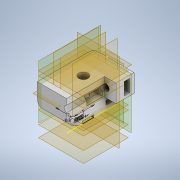
# Autodesk Inventor part: Encoder_Mount2
Saved by Autodesk Inventor 2022 (Build 260153000, 153)
## iProperties
Created: 2024-04-29
Part Number: Encoder_Mount2
Material: Generic
Document SubType Name: Modeling
Designer: Gotham City
Density: 1 g/cm^3
Appearance: Default
Author: Gotham City
Autodesk Inventor part; units mm, degrees
ref_plane "Alu_Top" through (0, 0, 0) normal (0, 1, 0) x (-1, 0, 0)
ref_plane "Strip" through (0, -20.8, 0) normal (0, 1, 0) x (-1, 0, 0)
ref_plane "Alu_Bottom" through (0, -2, 0) normal (0, 1, 0) x (-1, 0, 0)
ref_plane "EncoderPCB_Top" through (0, -25.8, 0) normal (0, 1, 0) x (-1, 0, 0)
ref_plane "Strip_V_End" through (5, 0, 0) normal (1, 0, 0) x (0, 1, 0)
ref_plane "Strip_V_Start" through (0, 0, 0) normal (1, 0, 0) x (0, 1, 0)
ref_plane "Encoder_PCB_Bottom" through (0, -15.2, 0) normal (0, 1, 0) x (-1, 0, 0)
ref_plane "Encoder_ScrewMount_V" through (-3.5, 0, 0) normal (1, 0, 0) x (0, 1, 0)
sketch "Sketch5" plane through (0, 0, 0) normal (0, 0, 1) x (1, 0, 0)
  line L0 (-7, -18.8) -> (5, -18.8)
  line L1 (5, -18.8) -> (5, -25.8)
  line L2 (5, -25.8) -> (-7, -25.8)
  line L3 (-7, -25.8) -> (-7, -18.8)
  line L4 (5, 5.06) -> (5, -30.36) construction
  line L5 (-9.4, -25.8) -> (7.4, -25.8) construction
  point P0 (0, 0)
  dimension "d10" = 12
  dimension "d11" = 7
  constraints: 8 end point, 2 parallel, 2 point on line, 1 horizontal, 1 perpendicular
  measures "d10" distance of L0.start L0.end
  measures "d11" distance of L0.end L1.end
extrude "Extrusion1" add sketch "Sketch5" along normal mid plane 7
sketch "Sketch6" plane through (-7, -25.8, 3.5) normal (0, -1, 0) x (1, 0, 0)
  line L0 (0, -12.5) -> (6.5, -12.5)
  line L1 (6.5, -12.5) -> (6.5, 5.5)
  line L2 (6.5, 5.5) -> (0, 5.5)
  line L3 (0, 5.5) -> (0, -12.5)
  line L4 (-2.4, -3.5) -> (14.4, -3.5) construction
  line L5 (3.5, 182.4494) -> (3.5, -189.4494) construction
  circle A0 centre (3.5, -10.5) radius 1
  line L6 (3.5, -189.4494) -> (3.5, 182.4494) construction
  circle A1 centre (3.5, 3.5) radius 1
  point P0 (7, -3.5)
  point P1 (0, -7)
  dimension "d14" = 18
  dimension "d15" = 6.5
  dimension "d16" = 14
  dimension "d17" = 2
  constraints: 10 end point, 3 point on line, 3 symmetric about line, 2 centre point, 2 parallel, 1 horizontal, 1 perpendicular, 2 other
  measures "d14" distance of L2.end L0.start
  measures "d15" distance of L0.start L0.end
  measures "d16" distance of A1.centre A0.centre
  measures "d17" diameter of A0
extrude "Extrusion2" add sketch "Sketch6" against normal up to surface (10.6 mm away)
sketch "Sketch4" plane through (0, 0, 0) normal (0, 0, 1) x (1, 0, 0)
  line L0 (-19.2812, -2) -> (9.0469, -2) construction
  line L1 (-8, -2) -> (5, -2)
  line L2 (5, -2) -> (5, -15.2)
  line L3 (5, -15.2) -> (-8, -15.2)
  line L4 (-8, -15.2) -> (-8, -2)
  line L5 (0, 3.75) -> (0, -22.5) construction
  line L6 (-8, -2) -> (-15.2344, -2) construction
  line L7 (-15.2344, -2) -> (-15.2344, -18.75) construction
  line L8 (-15.2344, -18.75) -> (-8, -18.75) construction
  line L9 (-8, -18.75) -> (-8, -2) construction
  line L10 (-19.2812, -15.2) -> (9.0469, -15.2) construction
  point P0 (0, 0)
  dimension "d54" = 5
  dimension "d55" = 8
  constraints: 16 end point, 4 parallel, 2 horizontal, 2 perpendicular, 2 point on line
  measures "d54" distance between parallel lines of L5 L2
  measures "d55" distance between parallel lines of L4 L5
extrude "Extrusion3" add sketch "Sketch4" along normal mid plane 25 separate body
ref_plane "SideA" through (0, 0, -12.5) normal (0, 0, -1) x (-1, 0, 0)
sketch "Sketch19" plane through (0, 0, -12.5) normal (0, 0, -1) x (-1, 0, 0)
  line L0 (-5, -2) -> (8, -2) projected
  line L1 (-5, -2) -> (-10, -2)
  line L2 (-10, -2) -> (-10, -10)
  line L3 (-10, -10) -> (-5, -10)
  line L4 (-5, -10) -> (-5, -2)
  point P0 (0, 0)
  dimension "d73" = 8
  dimension "d74" = 5
  constraints: 8 end point, 2 parallel, 1 horizontal, 1 perpendicular
  measures "d73" distance of L1.end L2.end
  measures "d74" distance of L0.start L1.end
extrude "Extrusion10" add sketch "Sketch19" against normal blind 8
sketch "Sketch7" plane through (0, 0, 0) normal (1, 0, 0) x (0, 1, 0)
  line L0 (-17.8, -3.5) -> (-17.8, 3.5) projected
  line L1 (-15.2, -12.5) -> (-15.2, 12.5) projected
  line L2 (-17.8, 3.5) -> (-15.2, 3.5)
  line L3 (-15.2, 3.5) -> (-15.2, -3.5)
  line L4 (-15.2, -3.5) -> (-17.8, -3.5)
  line L5 (-17.8, -3.5) -> (-17.8, 3.5)
  point P0 (0, 0)
  constraints: 8 end point, 2 parallel, 1 horizontal, 1 perpendicular, 1 point on line
extrude "Extrusion4" [suppressed]
sketch "Sketch8" plane through (0, -15.2, 0) normal (0, 1, 0) x (-1, 0, 0)
  circle A0 centre (3.5, 7) radius 1 projected
  circle A1 centre (3.5, -7) radius 1 projected
  point P0 (0, 0)
hole "Hole1" at (-3.5, -15.2, 7) at (-3.5, -15.2, -7) direction (0, 1, 0) diameter 2.1 depth 10 tip angle 118 clearance for "Socket Head Cap Screw ISO 4762" size "M2" standard "ISO"
ref_plane "Nut12" through (0, -13.2, 0) normal (0, 1, 0) x (-1, 0, 0)
sketch "Sketch10" plane through (0, -13.2, 0) normal (0, 1, 0) x (-1, 0, 0)
  circle A0 centre (3.5, 7) radius 1 construction
  line L0 (4.6691, 4.975) -> (2.3309, 4.975)
  line L1 (2.3309, 4.975) -> (1.1617, 7) construction
  line L2 (1.1617, 7) -> (2.3309, 9.025) construction
  line L3 (2.3309, 9.025) -> (4.6691, 9.025)
  line L4 (4.6691, 9.025) -> (5.8383, 7)
  line L5 (5.8383, 7) -> (4.6691, 4.975)
  line L6 (2.3309, 4.975) -> (-10, 4.975)
  line L7 (2.3309, 9.025) -> (-10, 9.025)
  line L8 (-10, 9.025) -> (-10, 4.975)
  line L9 (-10, -12.5) -> (-10, -4.5) projected
  point P0 (0, 0)
  dimension "d32" = 4.05
  constraints: 18 end point, 3 horizontal, 1 coincident, 1 perpendicular, 1 point on line, 13 other
  measures "d32" distance between parallel lines of L0 L3
extrude "Extrusion5" cut sketch "Sketch10" along normal blind 1.63
mirror "Mirror1" about plane through (0, 0, 0) normal (0, 0, 1) of "Extrusion5"
sketch "Sketch11" plane through (-8, -2, 12.5) normal (0, 1, 0) x (1, 0, 0)
  point P0 (8, 12.5)
  point P1 (8, 12.5)
  constraints: 1 coincident
hole "Hole2" at (0, -2, 0) direction (0, -1, 0) diameter 4.1 depth 8 tip angle 118 clearance for "Socket Head Cap Screw ISO 4762" size "M4" standard "ISO"
ref_plane "Nut3" through (-8, -6, 12.5) normal (0, 1, 0) x (1, 0, 0)
sketch "Sketch12" plane through (-8, -6, 12.5) normal (0, 1, 0) x (1, 0, 0)
  line L0 (3.9297, 12.5) -> (5.9648, 16.025)
  line L1 (5.9648, 16.025) -> (10.0352, 16.025)
  line L2 (10.0352, 16.025) -> (12.0703, 12.5) construction
  line L3 (12.0703, 12.5) -> (10.0352, 8.975) construction
  line L4 (10.0352, 8.975) -> (5.9648, 8.975)
  line L5 (5.9648, 8.975) -> (3.9297, 12.5)
  line L6 (10.0352, 16.025) -> (13, 16.025)
  line L7 (13, 17) -> (13, 0) projected
  line L8 (10.0352, 8.975) -> (13, 8.975)
  point P0 (8, 12.5)
  point P1 (8, 12.5)
  point P2 (13, 25)
  dimension "d45" = 7.05
  constraints: 16 end point, 2 horizontal, 2 point on line, 1 coincident, 1 parallel, 13 other
  measures "d45" distance between parallel lines of L1 L4
extrude "Extrusion6" cut sketch "Sketch12" against normal blind 3.25
sketch "Sketch13" plane through (0, 0, 0) normal (0, 0, 1) x (1, 0, 0)
  line L0 (-3, -19.8) -> (8, -19.8)
  line L1 (8, -19.8) -> (8, -21.8)
  line L2 (8, -21.8) -> (-3, -21.8)
  line L3 (-3, -21.8) -> (-3, -19.8)
  line L4 (0, 4.26) -> (0, -25.56) construction
  line L5 (5, 4.26) -> (5, -25.56) construction
  line L6 (-5.2, -20.8) -> (10.2, -20.8) construction
  point P0 (0, 0)
  dimension "d46" = 3
  dimension "d47" = 3
  dimension "d48" = 1
  dimension "d49" = 1
  constraints: 8 end point, 2 parallel, 1 horizontal, 1 perpendicular
  measures "d46" distance between parallel lines of L4 L3
  measures "d47" distance between parallel lines of L1 L5
  measures "d48" distance between parallel lines of L6 L0
  measures "d49" distance between parallel lines of L6 L2
extrude "Extrusion7" [suppressed]
ref_plane "EndstopScrew" through (0, -4.5, 0) normal (0, 1, 0) x (-1, 0, 0)
sketch "Sketch17" plane through (0, 0, -12.5) normal (0, 0, -1) x (-1, 0, 0)
  line L0 (-8.2, -6) -> (10.7, -6) projected
  point P0 (0, 0)
  point P1 (-5.5, -6)
  dimension "d60" = 5.5
  constraints: 1 point on line
  measures "d60" horizontal distance of point (0, 0) point (-5.5, -6)
hole "Hole3" at (5.5, -6, -12.5) direction (0, 0, 1) diameter 3 end through all clearance for "Socket Head Cap Screw ISO 4762" size "M3" standard "ISO"
ref_plane "Work Plane13" through (0, 0, -10.5) normal (0, 0, -1) x (-1, 0, 0)
sketch "Sketch18" plane through (0, 0, -10.5) normal (0, 0, -1) x (-1, 0, 0)
  circle A0 centre (-5.5, -6) radius 1.5 projected
  line L0 (-3.8979, -3.225) -> (-2.2957, -6)
  line L1 (-2.2957, -6) -> (-3.8979, -8.775)
  line L2 (-3.8979, -8.775) -> (-7.1021, -8.775)
  line L3 (-7.1021, -8.775) -> (-8.7043, -6) construction
  line L4 (-8.7043, -6) -> (-7.1021, -3.225) construction
  line L5 (-7.1021, -3.225) -> (-3.8979, -3.225)
  line L6 (-7.1021, -3.225) -> (-10, -3.225)
  line L7 (-7.1021, -8.775) -> (-10, -8.775)
  line L8 (-10, -10) -> (-10, -2) projected
  point P0 (0, 0)
  point P1 (-13, -14.8)
  point P2 (-10, -2)
  dimension "d69" = 5.55
  constraints: 16 end point, 4 horizontal, 2 coincident, 1 parallel, 16 other
  measures "d69" distance between parallel lines of L2 L5
extrude "Extrusion9" cut sketch "Sketch18" against normal blind 2.35
fillet "Fillet1" [suppressed]
thicken "Thicken1" [suppressed]
sketch "Sketch22" plane through (-3, -22.8, 3.5) normal (0, -1, 0) x (1, 0, 0)
  line L0 (-5, -16) -> (13, -16) projected
  line L1 (8, 9) -> (4, 9)
  line L2 (4, 9) -> (4, -16)
  line L3 (4, -16) -> (8, -16)
  line L4 (8, -16) -> (8, 9)
  line L5 (-5, 9) -> (-5, 0.1) projected
  circle A0 centre (-0.5, 3.5) radius 1.05 projected
  point P0 (3, -3.5)
  point P1 (8, 9)
  dimension "d84" = 4.5
  dimension "d85" = 4.5
  constraints: 8 end point, 2 parallel, 1 coincident, 1 horizontal, 1 midpoint, 1 perpendicular
  measures "d84" distance from line of L5 A0.centre
  measures "d85" distance from line of L2 A0.centre
extrude "Extrusion11" [suppressed]
ref_plane "Work Plane16" through (0, 0, -5) normal (0, 0, 1) x (1, 0, 0)
sketch "Sketch23" plane through (0, 0, -10.5) normal (0, 0, -1) x (-1, 0, 0)
  point P0 (0, 0)
sketch "Sketch24" plane through (-8, -15.2, 12.5) normal (-1, 0, 0) x (0, 0, 1)
  line L0 (-17.5, 20.36) -> (-17.5, -15.76) construction
  line L1 (-22, 5.2) -> (-13, 5.2) construction
  line L2 (-22, 4.15) -> (-13, 4.15)
  line L3 (-13, 6.25) -> (-22, 6.25)
  arc A0 (-22, 6.25) -> (-22, 4.15) centre (-22, 5.2) ccw
  arc A1 (-13, 4.15) -> (-13, 6.25) centre (-13, 5.2) ccw
  line L4 (-25, 13.2) -> (0, 13.2) projected
  point P0 (-12.5, 15.2)
  point P1 (-17.5, 5.2)
  dimension "d91" = 9
  dimension "d92" = 2.1
  dimension "d93" = 8
  constraints: 8 end point, 4 point on circle, 4 tangent, 2 centre point, 1 midpoint, 1 parallel, 1 perpendicular, 1 point on line
  measures "d91" distance of L1.start L1.end
  measures "d92" distance between parallel lines of L3 L2
  measures "d93" distance between parallel lines of L4 L1
ref_plane "Work Plane17" through (-6, -15.2, 12.5) normal (-1, 0, 0) x (0, 0, 1)
sketch "Sketch25" plane through (-6, -15.2, 12.5) normal (-1, 0, 0) x (0, 0, 1)
  line L0 (-25, 0) -> (-25, 13.2) projected
  line L1 (-25, 7.25) -> (-10.6329, 7.25)
  line L2 (-10.6329, 7.25) -> (-10.6329, 3.15)
  line L3 (-10.6329, 3.15) -> (-25, 3.15)
  line L4 (-25, 3.15) -> (-25, 7.25)
  line L5 (-25, 5.2) -> (-17, 5.2) projected
  line L6 (0, 0) -> (-25, 0) projected
  line L7 (0, 13.2) -> (0, 0) projected
  line L8 (-25, 13.2) -> (0, 13.2) projected
  line L9 (-25, 0) -> (-25, 13.2) projected
  line L10 (-11.8164, 3.15) -> (-14.1836, 3.15)
  line L11 (-14.1836, 3.15) -> (-15.3671, 5.2) construction
  line L12 (-15.3671, 5.2) -> (-14.1836, 7.25) construction
  line L13 (-14.1836, 7.25) -> (-11.8164, 7.25)
  line L14 (-11.8164, 7.25) -> (-10.6329, 5.2) construction
  line L15 (-10.6329, 5.2) -> (-11.8164, 3.15) construction
  point P0 (-12.5, 15.2)
  point P1 (-13, 5.2)
  point P2 (-13, 5.2)
  dimension "d95" = 4.1
  constraints: 20 end point, 2 horizontal, 2 parallel, 2 point on line, 1 coincident, 1 midpoint, 1 perpendicular, 14 other
  measures "d95" distance of L1.end L2.end
extrude "Extrusion12" [suppressed]
extrude "Extrusion13" [suppressed]
sketch "Sketch26" plane through (-8, -15.2, 12.5) normal (0, -1, 0) x (1, 0, 0)
  line L0 (8, -8) -> (1, -8)
  line L1 (1, -8) -> (1, -17)
  line L2 (1, -17) -> (8, -17)
  line L3 (8, -17) -> (8, -8)
  line L4 (4.5, -5.5) -> (4.5, -8) construction
  line L5 (4.5, -17) -> (4.5, -19.5) construction
  circle A0 centre (4.5, -5.5) radius 1.05 construction
  circle A1 centre (4.5, -19.5) radius 1.05 construction
  line L6 (13, -7) -> (8, -7)
  line L7 (8, -7) -> (8, -12)
  line L8 (8, -12) -> (13, -12)
  line L9 (13, -12) -> (13, -7)
  line L10 (13, -25) -> (13, 0) projected
  line L11 (8.8, -7) -> (8.8, -12)
  dimension "d106" = 9
  dimension "d107" = 7
  dimension "d114" = 1
  dimension "d115" = 4
  dimension "d116" = 0.8
  constraints: 22 end point, 4 parallel, 4 point on line, 3 perpendicular, 2 coincident, 2 horizontal, 2 midpoint, 2 vertical, 1 collinear
  measures "d106" distance of L2.end L0.start
  measures "d107" distance of L0.start L0.end
  measures "d114" distance from line of L0.start L6
  measures "d115" distance from line of L8 L0.start
  measures "d116" distance between parallel lines of L7 L11
extrude "Extrusion14" cut sketch "Sketch26" against normal blind 2 contours L3 L2 L1 L0
extrude "Extrusion15" cut sketch "Sketch26" against normal blind 1 contours L11 L6 L9 L8
chamfer "Chamfer2" distance 4 angle 45 1 edges at (-1.5, -15.2, 12.5)
fillet "Fillet3" radius 2 4 edges at (5, -12.6, -12.5) (5, -13.2, 10.5) (-8, -13.2, 10.5) (-8, -8.6, -12.5)
ref_plane "Screw" through (0, 0, 0) normal (1, 0, 0) x (0, 1, 0)
equation "\"d47\" = d46"
equation "\"d49\" = d48"
equation "\"d85\" = d84"
body "Solid1"
body "Solid2"
